Autodesk Inventor part; units mm, degrees
(part 3 of 3)
  spline S524 degree 2 poles (169.2646, -5.3029) (168.6665, -5.3029) (167.9398, -6.2075) (167.9398, -7.033) knots 0 0 0 1 2 2 2
  spline S525 degree 2 poles (167.9398, -7.033) (167.9398, -7.8388) (168.6418, -8.7434) (169.2646, -8.7434) knots 0 0 0 1 2 2 2
  spline S526 degree 2 poles (169.2646, -8.7434) (169.6403, -8.7434) (170.3225, -8.432) (170.5845, -8.1898) knots 0 0 0 1 2 2 2
  line L561 (170.5845, -8.1898) -> (170.629, -8.1898)
  line L562 (170.629, -8.1898) -> (170.629, -9.0548)
  spline S527 degree 2 poles (170.629, -9.0548) (170.5153, -9.1092) (170.1692, -9.2625) (170.0308, -9.2971) knots 0 0 0 1 2 2 2
  spline S528 degree 2 poles (170.0308, -9.2971) (169.8331, -9.3564) (169.5217, -9.4157) (169.2794, -9.4157) knots 0 0 0 1 2 2 2
  line L563 (175.1224, -9.3119) -> (174.109, -9.3119)
  line L564 (174.109, -9.3119) -> (172.4085, -7.1022)
  line L565 (172.4085, -7.1022) -> (172.1021, -7.3988)
  line L566 (172.1021, -7.3988) -> (172.1021, -9.3119)
  line L567 (172.1021, -9.3119) -> (171.3309, -9.3119)
  line L568 (171.3309, -9.3119) -> (171.3309, -2.94)
  line L569 (171.3309, -2.94) -> (172.1021, -2.94)
  line L570 (172.1021, -2.94) -> (172.1021, -6.6672)
  line L571 (172.1021, -6.6672) -> (173.9113, -4.7344)
  line L572 (173.9113, -4.7344) -> (174.8703, -4.7344)
  line L573 (174.8703, -4.7344) -> (172.9918, -6.6475)
  line L574 (172.9918, -6.6475) -> (175.1224, -9.3119)
  point P0 (0, 0)
  point P1 (-78.6298, -46.3653)
  point P2 (-78.6298, -46.3653)
  constraints: 26 other
extrude "EmbossedText" add sketch "Text" along normal blind 1
extrude "2mm_panel" add sketch "Cutouts" against normal blind 2 contours L0 L1 L2 L3 | L13 A8 | L14 A9
body "Solid3"
